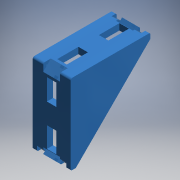
# Autodesk Inventor part: 14057_m
Saved by Autodesk Inventor 2019.4 (Build 234330000, 330)
## iProperties
Category: PARTsolutions
Company: 8020
Part Number: 14057_m
Material: ABS Plastic
Catalog Web Link: www.cadenas.de
Description: 14057, 14058_m-4 Hole Inside Corner Bracket
Vendor: 8020
Document SubType Name: Modeling
Designer: partserver
Manufacturer: 8020
Mass: 5.51644 g
Surface Area: 44.402 cm^2
Volume: 5.20419 cm^3
Density: 1.06 g/cm^3
Appearance: Cyan
PSOL_IDENT_0: {$CADENAS_DATA\23d-libs\8020\metric\joining_plates\14057_m.prj},160 {VTYP=3D},{NB=14057_m},{LINA=140
PSOL_IDENT_1: 57},{NN=14057, 14058_m},{DATE=31.07.2020 09:21:28},{GEOMDATE=09.09.2015 07:48:49},{VERSION=},{LINEID=
PSOL_IDENT_2: 10},{WBVAR=},{WBNUMERIC=}  {NB=14057_m},{LINA=14057},{KT=DUMMY},{PN=14057},{MAT=Die Cast Aluminum},{
PSOL_IDENT_3: FIN=Natural},{A=38.00},{B=18.00},{C=4.50},{D=5.00},{W=.013},{CC=5-20}
NB: 14057_m
NN: 14057, 14058_m
NT: 4 Hole Inside Corner Bracket
NBSYN: $PN._m
LINA: 14057
CATALOG: 80/20
PN: 14057
MAT: Die Cast Aluminum
FIN: Natural
A: 38
B: 18
C: 4.5
D: 5
W: .013
CC: 5-20
SUPPLIER: 8020
ARTICLENO: 14057_m
BOMINFO: 14057
CREATOR: CADENAS GmbH
Title: 14057
Author: Cadenas PARTsolutions
Comments: 4 Hole Inside Corner Bracket
Autodesk Inventor part; units mm, degrees
ref_plane "YZ Plane" through (0, 0, 0) normal (1, 0, 0) x (0, 1, 0)
ref_plane "XZ Plane" through (0, 0, 0) normal (0, 1, 0) x (-1, 0, 0)
ref_plane "XY Plane" through (0, 0, 0) normal (0, 0, 1) x (1, 0, 0)
sketch "Sketch1" plane through (9, 0, 0) normal (1, 0, 0) x (0, 0, -1)
  line L0 (-38, 0.5) -> (-37.5, 0)
  line L1 (-37.5, 0) -> (-1, 0)
  arc A0 (-1, 0) -> (0, 1) centre (-1, 1) ccw
  line L2 (0, 1) -> (0, 37.5)
  line L3 (0, 37.5) -> (-0.5, 38)
  line L4 (-0.5, 38) -> (-2.5, 38)
  line L5 (-2.5, 38) -> (-38, 2.5)
  line L6 (-38, 2.5) -> (-38, 0.5)
  constraints: 14 end point, 2 point on circle, 1 centre point
extrude "Extrusion1" add sketch "Sketch1" against normal blind 18
sketch "Sketch4" plane through (9, 0, 0) normal (1, 0, 0) x (0, 0, -1)
  line L0 (-37.5, 3) -> (-3.5, 3)
  arc A0 (-3.5, 3) -> (-3, 3.5) centre (-3.5, 3.5) ccw
  line L1 (-3, 3.5) -> (-3, 37.5)
  line L2 (-3, 37.5) -> (-37.5, 3)
  constraints: 6 end point, 2 point on circle, 1 centre point
extrude "Extrusion2" cut sketch "Sketch4" against normal blind 15
sketch "Sketch7" plane through (4.5, 0, 0) normal (-1, 0, 0) x (0, -1, 0)
  line L0 (-5.8284, 3) -> (-3.5, 3)
  arc A0 (-3.5, 3) -> (-3, 3.5) centre (-3.5, 3.5) ccw
  line L1 (-3, 3.5) -> (-3, 5.8284)
  line L2 (-3, 5.8284) -> (-5.8284, 3)
  constraints: 6 end point, 2 point on circle, 1 centre point
extrude "Extrusion3" add sketch "Sketch7" against normal blind 3
sketch "Sketch10" plane through (4, 0, 0) normal (1, 0, 0) x (0, 0, -1)
  line L0 (-1.4142, 36.0858) -> (0, 34.6716)
  line L1 (0, 34.6716) -> (0, 37.5)
  line L2 (0, 37.5) -> (-1.4142, 36.0858)
  constraints: 6 end point
extrude "Extrusion4" cut sketch "Sketch10" against normal blind 8
sketch "Sketch13" plane through (4, 0, 0) normal (1, 0, 0) x (0, 0, -1)
  line L0 (-37.5, 0) -> (-34.6716, 0)
  line L1 (-34.6716, 0) -> (-36.0858, 1.4142)
  line L2 (-36.0858, 1.4142) -> (-37.5, 0)
  constraints: 6 end point
extrude "Extrusion5" cut sketch "Sketch13" against normal blind 8
sketch "Sketch16" plane through (4, 0, 0) normal (-1, 0, 0) x (0, 0, 1)
  line L0 (35.5, 0) -> (37.5, 0)
  line L1 (37.5, 0) -> (38, 0.5)
  line L2 (38, 0.5) -> (38, 2.0977)
  line L3 (38, 2.0977) -> (35.5, 0)
  constraints: 8 end point
extrude "Extrusion6" cut sketch "Sketch16" against normal blind 3
sketch "Sketch19" plane through (-4, 0, 0) normal (1, 0, 0) x (0, 0, -1)
  line L0 (-2.0977, 38) -> (0, 35.5)
  line L1 (0, 35.5) -> (0, 37.5)
  line L2 (0, 37.5) -> (-0.5, 38)
  line L3 (-0.5, 38) -> (-2.0977, 38)
  constraints: 8 end point
extrude "Extrusion7" cut sketch "Sketch19" against normal blind 3
sketch "Sketch22" plane through (4, 0, 0) normal (-1, 0, 0) x (0, 0, 1)
  line L0 (0, 37.5) -> (0, 35.5)
  line L1 (0, 35.5) -> (2.0977, 38)
  line L2 (2.0977, 38) -> (0.5, 38)
  line L3 (0.5, 38) -> (0, 37.5)
  constraints: 8 end point
extrude "Extrusion8" cut sketch "Sketch22" against normal blind 3
sketch "Sketch25" plane through (-4, 0, 0) normal (1, 0, 0) x (0, 0, -1)
  line L0 (-38, 0.5) -> (-37.5, 0)
  line L1 (-37.5, 0) -> (-35.5, 0)
  line L2 (-35.5, 0) -> (-38, 2.0977)
  line L3 (-38, 2.0977) -> (-38, 0.5)
  constraints: 8 end point
extrude "Extrusion9" cut sketch "Sketch25" against normal blind 3
sketch "Sketch28" plane through (4, 0, 0) normal (1, 0, 0) x (0, 0, -1)
  line L0 (-3.677, 0) -> (-1, 0)
  arc A0 (-1, 0) -> (0, 1) centre (-1, 1) ccw
  line L1 (0, 1) -> (0, 3.677)
  line L2 (0, 3.677) -> (-1.6617, 2.0153)
  line L3 (-1.6617, 2.0153) -> (-1.3081, 1.6617)
  line L4 (-1.3081, 1.6617) -> (-1.6617, 1.3081)
  line L5 (-1.6617, 1.3081) -> (-2.0153, 1.6617)
  line L6 (-2.0153, 1.6617) -> (-3.677, 0)
  constraints: 14 end point, 2 point on circle, 1 centre point
extrude "Extrusion10" cut sketch "Sketch28" against normal blind 8
sketch "Sketch43" plane through (2.25, 0, 0) normal (1, 0, 0) x (0, 0, -1)
  line L0 (-15, 0) -> (-4.9497, 0)
  line L1 (-4.9497, 0) -> (-7.9497, 3)
  line L2 (-7.9497, 3) -> (-15, 3)
  line L3 (-15, 3) -> (-15, 0)
  constraints: 8 end point
extrude "Extrusion11" cut sketch "Sketch43" against normal blind 4.5
sketch "Sketch46" plane through (2.25, 0, 0) normal (1, 0, 0) x (0, 0, -1)
  line L0 (-3, 27.7487) -> (0, 24.7487)
  line L1 (0, 24.7487) -> (0, 34.5)
  line L2 (0, 34.5) -> (-3, 34.5)
  line L3 (-3, 34.5) -> (-3, 27.7487)
  constraints: 8 end point
extrude "Extrusion12" cut sketch "Sketch46" against normal blind 4.5
sketch "Sketch49" plane through (2.25, 0, 0) normal (1, 0, 0) x (0, 0, -1)
  line L0 (-3, 7.9497) -> (0, 4.9497)
  line L1 (0, 4.9497) -> (0, 15)
  line L2 (0, 15) -> (-3, 15)
  line L3 (-3, 15) -> (-3, 7.9497)
  constraints: 8 end point
extrude "Extrusion13" cut sketch "Sketch49" against normal blind 4.5
sketch "Sketch52" plane through (2.25, 0, 0) normal (1, 0, 0) x (0, 0, -1)
  line L0 (-34.5, 0) -> (-24.7487, 0)
  line L1 (-24.7487, 0) -> (-27.7487, 3)
  line L2 (-27.7487, 3) -> (-34.5, 3)
  line L3 (-34.5, 3) -> (-34.5, 0)
  constraints: 8 end point
extrude "Extrusion14" cut sketch "Sketch52" against normal blind 4.5
sketch "Sketch_1" plane through (0, 0, 0) normal (1, 0, 0) x (0, 1, 0)
  line L0 (0.0707, 3.6062) -> (-1.4849, 2.0506)
  line L1 (-1.4849, 2.0506) -> (-0.7778, 1.3435)
  line L2 (-0.7778, 1.3435) -> (0.7778, 2.8991)
  line L3 (0.7778, 2.8991) -> (0.0707, 3.6062)
  constraints: 8 end point
sketch "Sketch_2" plane through (0, 0, 0) normal (1, 0, 0) x (0, 1, 0)
  line L0 (2.8991, 0.7778) -> (1.3435, -0.7778)
  line L1 (1.3435, -0.7778) -> (2.0506, -1.4849)
  line L2 (2.0506, -1.4849) -> (3.6062, 0.0707)
  line L3 (3.6062, 0.0707) -> (2.8991, 0.7778)
  constraints: 8 end point
extrude "Extrusion15" add sketch "Sketch_1" along normal mid plane 5
extrude "Extrusion16" add sketch "Sketch_2" along normal mid plane 5
sketch "Sketch_3" plane through (0, 0, 0) normal (1, 0, 0) x (0, 1, 0)
  line L0 (36.7929, 0.7071) -> (35.308, -0.7778)
  line L1 (35.308, -0.7778) -> (36.0151, -1.4849)
  line L2 (36.0151, -1.4849) -> (37.5, 0)
  line L3 (37.5, 0) -> (36.7929, 0.7071)
  constraints: 8 end point
sketch "Sketch_4" plane through (0, 0, 0) normal (1, 0, 0) x (0, 1, 0)
  line L0 (0, 37.5) -> (-1.4849, 36.0151)
  line L1 (-1.4849, 36.0151) -> (-0.7778, 35.308)
  line L2 (-0.7778, 35.308) -> (0.7071, 36.7929)
  line L3 (0.7071, 36.7929) -> (0, 37.5)
  constraints: 8 end point
extrude "Extrusion17" add sketch "Sketch_3" along normal mid plane 5
extrude "Extrusion18" add sketch "Sketch_4" along normal mid plane 5
body "Solid1"
